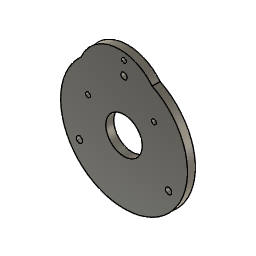
Generator mount (Autodesk Fusion 360 design; units mm, degrees)
part number: 2025-06-12-14-02-21-986
Autodesk Fusion 360 part; units mm, degrees
note: some values were not read from the file. Set by a fixed rule: which sketch regions a step uses.
sketch "Sketch2" plane through (0, 0, 0) normal (0, 1, 0) x (1, 0, 0)
  circle A0 centre (0, 0) radius 80
  circle A1 centre (0, -65) radius 4
  circle A2 centre (-56.2917, 32.5) radius 4
  circle A3 centre (56.2917, 32.5) radius 4
  circle A4 centre (0, 0) radius 23
  dimension "d29" = 160
  dimension "d30" = 8
  dimension "d31" = 8
  dimension "d32" = 8
  dimension "d33" = 120
  dimension "d34" = 120
  dimension "d35" = 65
  dimension "d36" = 65
  dimension "d37" = 65
  dimension "d38" = 46
  constraint coincident A0.centre A4.centre
  measures "d29" diameter of A0
  measures "d30" diameter of A1
  measures "d31" diameter of A2
  measures "d32" diameter of A3
  measures "d33" angle of A0.centre A1.centre A2.centre
  measures "d34" angle of A0.centre A1.centre A3.centre
  measures "d35" distance of A0.centre A3.centre
  measures "d36" distance of A0.centre A2.centre
  measures "d37" distance of A0.centre A1.centre
  measures "d38" diameter of A4
sketch "Sketch3" plane through (0, 0, 0) normal (0, 1, 0) x (1, 0, 0)
  circle A0 centre (0, -82) radius 3
  circle A1 centre (0, -65) radius 4
  circle A2 centre (37.7308, -33.7512) radius 3
  circle A3 centre (-45.463, -21.7852) radius 3
  circle A4 centre (-5.4604, -38.8527) radius 43.4915 construction
  line L0 (0, 0) -> (0, -106.7199)
  line L1 (0, 0) -> (-5.4604, -38.8527) construction
  circle A5 centre (-5.4604, -38.8527) radius 52.5
  line L2 (-44.0663, -23.3245) -> (-50.9, -23.3245)
  line L3 (-47.433, -26.5975) -> (-47.433, -19.6919)
  line L4 (32.8029, -32.5277) -> (40.5, -32.5277)
  line L5 (36.1117, -35.7471) -> (36.1117, -28.3628)
  point P0 (-47.433, -23.3245)
  point P1 (36.1117, -32.5277)
  dimension "d40" = 6
  dimension "d41" = 17
  dimension "d42" = 6
  dimension "d43" = 61.25
  dimension "d44" = 6
  dimension "d45" = 84.05
  dimension "d46" = 75.45
  dimension "d47" = 8
  dimension "d48" = 105
  constraint coincident A0.centre A4
  constraint coincident A2.centre A4
  constraint coincident A3.centre A4
  constraint coincident L0.start L1.start
  constraint vertical L0
  constraint coincident A4.centre L1.end
  constraint concentric A4 A5
  constraint horizontal L2
  constraint perpendicular L2 L3
  constraint horizontal L4
  constraint perpendicular L4 L5
  constraint coincident L3 P0
  constraint coincident L2 P0
  constraint coincident L5 P1
  constraint coincident L4 P1
  measures "d40" diameter of A0
  measures "d41" distance of A0.centre A1.centre
  measures "d42" diameter of A2
  measures "d43" distance of A0.centre A2.centre
  measures "d44" diameter of A3
  measures "d45" distance of A2.centre A3.centre
  measures "d46" distance of A0.centre A3.centre
  measures "d47" angle of L0 L1
  measures "d48" diameter of A5
extrude "Extrude1" add sketch "Sketch3" sketch "Sketch2" along normal blind 10 of sketch 2
extrude "Extrude2" cut sketch "Sketch3" along normal blind 10 contours A0 L0 | A0 L0
extrude "Extrude3" cut sketch "Sketch2" along normal blind 10 contours A4
extrude "Extrude4" cut sketch "Sketch3" along normal blind 10 contours A3 L2 L3 | A3 L2 L3
extrude "Extrude5" cut sketch "Sketch3" along normal blind 10 contours A2 L4 | A2 L4 L5 | A2 L4 L5
sketch "Sketch4" plane through (0, 0, 0) normal (0, -1, 0) x (1, 0, 0)
  circle A0 centre (37.7308, 33.7512) radius 3
  circle A1 centre (-45.463, 21.7852) radius 3
  circle A2 centre (0, 65) radius 4
  circle A3 centre (0, 0) radius 23
  circle A4 centre (56.2917, -32.5) radius 4
  circle A5 centre (-56.2917, -32.5) radius 4
  arc A6 (35.5015, 71.6913) -> (-53.887, 59.1286) centre (-5.4604, 38.8527) ccw
  arc A7 (-53.887, 59.1286) -> (35.5015, 71.6913) centre (0, 0) ccw
  circle A8 centre (0, 82) radius 3
  circle A9 centre (0, 0) radius 23
  circle A10 centre (37.7308, 33.7512) radius 3
  circle A11 centre (0, 65) radius 4
  circle A12 centre (0, 82) radius 3
  circle A13 centre (-45.463, 21.7852) radius 3
  circle A14 centre (-56.2917, -32.5) radius 4
  circle A15 centre (56.2917, -32.5) radius 4
  line L0 (0, 83.5) -> (0, 80)
  line L1 (-1.6, 82) -> (1.6, 82)
  line L2 (0, 67.3) -> (0, 62.5)
  line L3 (-3, 65) -> (3.4, 65)
  line L4 (35.496, 33.7512) -> (39.8, 33.7512)
  line L5 (37.7308, 36.0039) -> (37.7308, 31.5)
  line L6 (-45.463, 24.0048) -> (-45.463, 19.2402)
  line L7 (-47.6513, 21.7852) -> (-43.1669, 21.7852)
  line L8 (-56.2917, -29.4965) -> (-56.2917, -35.5)
  line L9 (-59, -32.5) -> (-53.5, -32.5)
  line L10 (56.2917, -29.0015) -> (56.2917, -36)
  line L11 (53.1873, -32.5) -> (59.5, -32.5)
  line L12 (0, 10) -> (0, -9.5078)
  line L13 (-10, 0) -> (10, 0)
  dimension "d59" = 46
  dimension "d60" = 6
  dimension "d61" = 8
  dimension "d62" = 6
  dimension "d63" = 6
  dimension "d64" = 8
  dimension "d65" = 8
  constraint concentric A0 A10
  constraint concentric A2 A11
  constraint concentric A8 A12
  constraint concentric A1 A13
  constraint concentric A5 A14
  constraint concentric A4 A15
  constraint coincident A3.centre A7.centre
  constraint vertical L0
  constraint perpendicular L0 L1
  constraint vertical L2
  constraint perpendicular L2 L3
  constraint horizontal L4
  constraint perpendicular L4 L5
  constraint vertical L6
  constraint perpendicular L6 L7
  constraint vertical L8
  constraint perpendicular L8 L9
  constraint vertical L10
  constraint perpendicular L10 L11
  constraint vertical L12
  constraint perpendicular L12 L13
  measures "d59" diameter of A9
  measures "d60" diameter of A10
  measures "d61" diameter of A11
  measures "d62" diameter of A12
  measures "d63" diameter of A13
  measures "d64" diameter of A14
  measures "d65" diameter of A15
